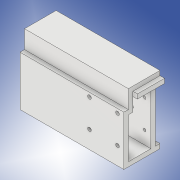
# Autodesk Inventor part: FA003
Saved by Autodesk Inventor 2017 SP1 (Build 210196100, 196)
## iProperties
Created: 2017-06-16
Part Number: FA003
Material: ABS Plastic
Document SubType Name: Modeling
Designer: Zach
Density: 1.06 g/cm^3
Appearance: CR White
Author: Zach
Autodesk Inventor part; units mm, degrees
ref_plane "YZ Plane" through (0, 0, 0) normal (1, 0, 0) x (0, 1, 0)
ref_plane "XZ Plane" through (0, 0, 0) normal (0, 1, 0) x (-1, 0, 0)
sketch "Sketch1" plane through (0, 0, 0) normal (0, 0, 1) x (1, 0, 0)
  line L0 (0, 0) -> (115, 0)
  line L1 (115, 0) -> (115, 75)
  line L2 (115, 75) -> (0, 75)
  line L3 (0, 75) -> (0, 0)
  dimension "d0" = 115
  dimension "d1" = 75
  constraints: 8 end point, 2 parallel, 1 horizontal, 1 perpendicular
  measures "d0" distance of L2.end L1.end
  measures "d1" distance of L1.end L0.end
extrude "Extrusion1" add sketch "Sketch1" along normal blind 40
sketch "Sketch2" plane through (0, 0, 40) normal (0, 0, 1) x (1, 0, 0)
  line L0 (115, 75) -> (0, 75) projected
  line L1 (115, 0) -> (115, 75) projected
  line L2 (0, 75) -> (115, 75)
  line L3 (115, 75) -> (115, 55)
  line L4 (115, 55) -> (0, 55)
  line L5 (0, 55) -> (0, 75)
  point P0 (0, 0)
  dimension "d4" = 20
  constraints: 8 end point, 2 parallel, 1 horizontal, 1 perpendicular, 1 point on line
  measures "d4" distance of L2.end L3.end
extrude "Extrusion2" cut sketch "Sketch2" against normal blind 5
sketch "Sketch3" plane through (115, 0, 0) normal (1, 0, 0) x (0, 0, -1)
  line L0 (0, 75) -> (-35, 75) projected
  line L1 (-35, 75) -> (-35, 55) projected
  line L2 (-35, 55) -> (-40, 55) projected
  line L3 (-40, 0) -> (-40, 55) projected
  line L4 (0, 0) -> (-40, 0) projected
  line L5 (0, 70) -> (-30, 70)
  line L6 (-30, 70) -> (-30, 50)
  line L7 (-30, 50) -> (-35, 50)
  line L8 (-35, 50) -> (-35, 5)
  line L9 (-35, 5) -> (0, 5)
  line L10 (0, 5) -> (0, 70)
  line L11 (0, 0) -> (0, 75) projected
  dimension "d7" = 5
  constraints: 12 end point, 1 collinear, 4 other
  measures "d7" distance between parallel lines of L0 L5
extrude "Extrusion3" cut sketch "Sketch3" against normal through all contours L10 L9 L8 L7 L6 L5
sketch "Sketch11" plane through (0, 0, 0) normal (0, 0, -1) x (-1, 0, 0)
  line L0 (-120, 70) -> (5, 70)
  line L1 (5, 70) -> (5, 65)
  line L2 (5, 65) -> (-120, 65)
  line L3 (-120, 65) -> (-120, 70)
  line L4 (-115, 70) -> (-115, 75) projected
  point P0 (0, 0)
  point P1 (0, 70)
  dimension "d42" = 5
  dimension "d43" = 5
  dimension "d44" = 5
  constraints: 8 end point, 2 parallel, 1 horizontal, 1 horizontal alignment, 1 perpendicular
  measures "d42" distance of L0.end L1.end
  measures "d43" distance of L0.end point (0, 70)
  measures "d44" distance from line of L4 L0.start
extrude "Extrusion11" add sketch "Sketch11" against normal blind 30
ref_plane "Work Plane2" through (0, 0, 5) normal (0, 0, -1) x (-1, 0, 0)
sketch "Sketch12" plane through (0, 0, 5) normal (0, 0, -1) x (-1, 0, 0)
  line L0 (-115, 50) -> (-115, 65)
  line L1 (-115, 5) -> (0, 5)
  line L2 (-115, 65) -> (-70, 65)
  line L3 (-70, 65) -> (-70, 5)
  line L4 (-70, 5) -> (-115, 5)
  line L5 (-115, 5) -> (-115, 65)
  line L6 (-108, 50.5) -> (-77, 50.5) construction
  line L7 (-77, 50.5) -> (-77, 19.5) construction
  line L8 (-77, 19.5) -> (-108, 19.5) construction
  line L9 (-108, 19.5) -> (-108, 50.5) construction
  circle A0 centre (-77, 50.5) radius 1.5
  circle A1 centre (-108, 50.5) radius 1.5
  circle A2 centre (-77, 19.5) radius 1.5
  circle A3 centre (-108, 19.5) radius 1.5
  circle A4 centre (-92.5, 35) radius 3
  point P0 (0, 0)
  point P1 (-5, 5)
  point P2 (-92.5, 50.5)
  point P3 (-92.5, 65)
  point P4 (-108, 35)
  point P5 (-115, 35)
  dimension "d47" = 45
  dimension "d48" = 31
  dimension "d49" = 31
  dimension "d50" = 3
  dimension "d51" = 3
  dimension "d52" = 3
  dimension "d53" = 3
  dimension "d54" = 6
  constraints: 20 end point, 5 centre point, 4 coincident, 4 midpoint, 4 parallel, 2 horizontal, 2 horizontal alignment, 2 perpendicular, 2 vertical alignment, 1 point on line
  measures "d47" distance of L3.end L4.end
  measures "d48" distance of L7.end L8.end
  measures "d49" distance of L6.end L7.end
  measures "d50" diameter of A0
  measures "d51" diameter of A1
  measures "d52" diameter of A2
  measures "d53" diameter of A3
  measures "d54" diameter of A4
extrude "Extrusion12" add sketch "Sketch12" against normal blind 5
sketch "Sketch13" plane through (0, 0, 5) normal (0, 0, -1) x (-1, 0, 0)
  circle A0 centre (-92.5, 35) radius 3
  circle A1 centre (-92.5, 35) radius 12.5
  point P0 (0, 0)
  dimension "d57" = 25
  constraints: 2 centre point, 1 coincident
  measures "d57" diameter of A1
extrude "Extrusion13" cut sketch "Sketch13" against normal blind 2
sketch "Sketch15" plane through (0, 0, 10) normal (0, 0, 1) x (1, 0, 0)
  circle A0 centre (108, 50.5) radius 1.5 projected
  circle A1 centre (108, 19.5) radius 1.5 projected
  circle A2 centre (77, 50.5) radius 1.5 projected
  circle A3 centre (77, 19.5) radius 1.5 projected
  circle A4 centre (77, 50.5) radius 2
  circle A5 centre (108, 50.5) radius 2
  circle A6 centre (108, 19.5) radius 2
  circle A7 centre (77, 19.5) radius 2
  point P0 (0, 0)
  dimension "d60" = 4
  dimension "d61" = 4
  dimension "d62" = 4
  dimension "d63" = 4
  constraints: 4 centre point, 4 coincident
  measures "d60" diameter of A4
  measures "d61" diameter of A5
  measures "d62" diameter of A6
  measures "d63" diameter of A7
extrude "Extrusion14" cut sketch "Sketch15" along normal through all contours A0 | A1 | A2 | A3 | A4 | A5 | A6 | A7
sketch "Sketch16" plane through (115, 5, 35) normal (0, 0, -1) x (-1, 0, 0)
  circle A0 centre (85, 25) radius 10
  circle A1 centre (85, 25) radius 2.5
  line L0 (115, 45) -> (115, 0) projected
  line L1 (115, -5) -> (0, -5) projected
  dimension "d66" = 20
  dimension "d67" = 5
  dimension "d68" = 30
  dimension "d69" = 30
  constraints: 2 centre point, 1 coincident
  measures "d66" diameter of A0
  measures "d67" diameter of A1
  measures "d68" distance from line of L0 A0.centre
  measures "d69" distance from line of L1 A0.centre
extrude "Extrusion15" add sketch "Sketch16" along normal blind 35
body "Solid1"
